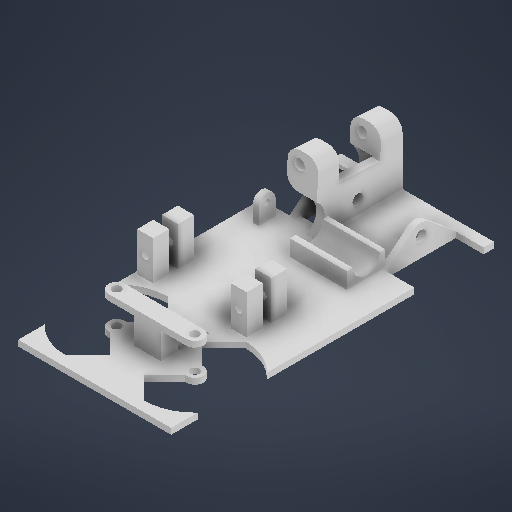
# Autodesk Inventor part: Рама
Saved by Autodesk Inventor 2026.2 (Build 302298000, 298)
## iProperties
Created: 2026-02-19
Part Number: Рама
Material: Типовые
Document SubType Name: Modeling
Designer: Leonid
Density: 1 g/cm^3
Appearance: По умолчанию
Author: Leonid
Autodesk Inventor part; units mm, degrees
ref_plane "XZ Plane" through (0, 0, 0) normal (0, 1, 0) x (-1, 0, 0)
ref_plane "XY Plane" through (0, 0, 0) normal (0, 0, 1) x (1, 0, 0)
sketch "Эскиз1" plane through (0, 0, 0) normal (0, 1, 0) x (-1, 0, 0)
  line L0 (-22.5, -47.5) -> (22.5, -47.5)
  line L1 (22.5, -47.5) -> (22.5, 14.5)
  line L2 (22.5, 47.5) -> (-22.5, 47.5)
  line L3 (-22.5, 47.5) -> (-22.5, 44.5)
  line L4 (-22.5, -47.5) -> (22.5, 47.5) construction
  line L5 (22.5, -47.5) -> (-22.5, 47.5) construction
  line L6 (22.5, 29.5) -> (-22.5, 29.5) construction
  line L7 (-22.5, 44.5) -> (-22.5, 14.5)
  line L8 (-22.5, 14.5) -> (-22.5, -47.5)
  line L9 (22.5, 14.5) -> (22.5, 44.5)
  line L10 (22.5, 44.5) -> (22.5, 47.5)
  circle A0 centre (11.5, 29.5) radius 1.325
  line L11 (22.5, 44.5) -> (5, 44.5)
  line L12 (-22.5, 44.5) -> (-5, 44.5)
  arc A1 (11.5, 27) -> (11.5, 32) centre (11.5, 29.5) ccw
  line L13 (11.5, 32) -> (5, 32)
  circle A2 centre (-11.5, 29.5) radius 1.325
  arc A3 (-11.5, 32) -> (-11.5, 27) centre (-11.5, 29.5) ccw
  line L14 (-11.5, 32) -> (-5, 32)
  line L15 (11.5, 27) -> (-11.5, 27)
  line L16 (22.5, 14.5) -> (-22.5, 14.5)
  line L17 (5, 32) -> (5, 44.5)
  line L18 (-5, 32) -> (-5, 44.5)
  line L19 (-11.5, 44.5) -> (-5, 38)
  line L20 (-11.5, 44.5) -> (-2.3076, 44.5) construction
  line L21 (11.5, 44.5) -> (5, 38)
  line L22 (11.5, 44.5) -> (20.6924, 44.5) construction
  line L23 (5, 38) -> (11, 32)
  line L24 (-5, 38) -> (-11, 32)
  arc A4 (-11.5, 44.5) -> (-22.5, 39.698) centre (-11.5, 29.5) ccw
  arc A5 (22.5, 39.698) -> (11.5, 44.5) centre (11.5, 29.5) ccw
  arc A6 (-22.5, 19.302) -> (-11.5, 14.5) centre (-11.5, 29.5) ccw
  arc A7 (11.5, 14.5) -> (22.5, 19.302) centre (11.5, 29.5) ccw
  line L25 (-11.5, 44.5) -> (-11.5, 14.5) construction
  line L26 (11.5, 44.5) -> (11.5, 14.5) construction
  line L27 (-11, 27) -> (-5, 21)
  line L28 (-11, 27) -> (-2.5147, 27) construction
  line L29 (-5, 21) -> (-11.5, 14.5)
  line L30 (11.5, 14.5) -> (5, 21)
  line L31 (11.5, 14.5) -> (20.6924, 14.5) construction
  line L32 (5, 21) -> (11, 27)
  line L33 (-5.8, 8.55) -> (-10.55, 8.55)
  line L34 (-10.55, 8.55) -> (-10.55, 13.3)
  line L35 (-10.55, 13.3) -> (-5.8, 13.3)
  line L36 (-5.8, 13.3) -> (-5.8, 8.55)
  line L37 (16.95, 8.55) -> (21.7, 8.55)
  line L38 (21.7, 8.55) -> (21.7, 13.3)
  line L39 (21.7, 13.3) -> (16.95, 13.3)
  line L40 (16.95, 13.3) -> (16.95, 8.55)
  line L41 (-5.8, 1.3) -> (-10.55, 1.3)
  line L42 (-10.55, 1.3) -> (-10.55, 6.05)
  line L43 (-10.55, 6.05) -> (-5.8, 6.05)
  line L44 (-5.8, 6.05) -> (-5.8, 1.3)
  line L45 (16.95, 1.3) -> (21.7, 1.3)
  line L46 (21.7, 1.3) -> (21.7, 6.05)
  line L47 (21.7, 6.05) -> (16.95, 6.05)
  line L48 (16.95, 6.05) -> (16.95, 1.3)
  line L49 (22.5, -44.5) -> (-22.5, -44.5)
  line L50 (-22.5, -24.104) -> (-14.25, -24.104)
  line L51 (-14.25, -24.104) -> (-14.25, -44.5)
  line L52 (22.5, -24.104) -> (14.25, -24.104)
  line L53 (14.25, -24.104) -> (14.25, -44.5)
  line L54 (7, -25.63) -> (12.5, -25.63)
  line L55 (12.5, -25.63) -> (12.5, -42.974)
  line L56 (12.5, -42.974) -> (7, -42.974)
  line L57 (7, -42.974) -> (7, -25.63)
  line L58 (-7.8, 13.3) -> (16.95, 13.3)
  line L59 (16.95, 13.3) -> (16.95, -11.2)
  line L60 (16.95, -11.2) -> (-7.8, -11.2)
  line L61 (-7.8, -11.2) -> (-7.8, 13.3)
  line L62 (-4, 27) -> (4, 27)
  line L63 (4, 27) -> (4, 32)
  line L64 (4, 32) -> (-4, 32)
  line L65 (-4, 32) -> (-4, 27)
  line L66 (-4, 27) -> (4, 32) construction
  line L67 (4, 27) -> (-4, 32) construction
  line L68 (12.5, -34.302) -> (14.25, -34.302) construction
  point P0 (0, 0)
  point P1 (13.75, 44.5)
  point P2 (-12.5, -44.5)
  point P3 (-7.8, 1.3)
  point P4 (16.95, 1.3)
  point P5 (-7.8, 8.55)
  point P6 (-7.8, 6.05)
  point P7 (0, 29.5)
  point P8 (-4, 27)
  point P9 (4, 27)
  dimension "d0" = 45
  dimension "d6" = 3
  dimension "d7" = 2.65
  dimension "d8" = 11
  dimension "d14" = 2.65
  dimension "d15" = 11
  dimension "d16" = 2.5
  dimension "d19" = 10
  dimension "d20" = 12.5
  dimension "d22" = 95
  dimension "d23" = 12.5
  dimension "d25" = 23
  dimension "d26" = 45
  dimension "d27" = 135
  dimension "d29" = 23
  dimension "d30" = 45
  dimension "d31" = 135
  dimension "d37" = 0.5
  dimension "d38" = 32.25
  dimension "d39" = 22.75
  dimension "d40" = 4.75
  dimension "d42" = 5.95
  dimension "d43" = 32.25
  dimension "d44" = 22.75
  dimension "d45" = 4.75
  dimension "d46" = 2.5
  dimension "d60" = 20.3961
  dimension "d61" = 3
  dimension "d62" = 20.396
  dimension "d63" = 8.25
  dimension "d70" = 5.55
  dimension "d72" = 5.5
  dimension "d73" = 17.344
  dimension "d101" = 24.5
  dimension "d102" = 2
  dimension "d120" = 8
  dimension "d123" = 1.75
  constraints: 138 end point, 31 point on line, 23 perpendicular, 22 parallel, 17 horizontal, 12 point on circle, 11 equal length, 10 midpoint, 8 centre point, 6 coincident, 6 collinear, 6 tangent, 1 vertical
  measures "d0" distance of L2.end L2.start
  measures "d6" distance of L9.end L2.start
  measures "d7" diameter of A0
  measures "d8" distance from line of A0.centre L9
  measures "d14" diameter of A2
  measures "d15" distance from line of L7 A2.centre
  measures "d16" radius of A3
  measures "d19" distance between parallel lines of L18 L17
  measures "d20" distance between parallel lines of L16 L15
  measures "d22" distance between parallel lines of L0 L2
  measures "d23" vertical distance of L3.end L14.start
  measures "d25" distance of A2.centre A0.centre
  measures "d26" angle of L19 L20
  measures "d27" angle of L21 L22
  measures "d29" distance of L19.start L21.start
  measures "d30" angle of L27 L28
  measures "d31" angle of L31 L30
  measures "d37" distance of L15.start L32.end
  measures "d38" distance between parallel lines of L34 L38
  measures "d39" distance between parallel lines of L36 L40
  measures "d40" distance between parallel lines of L35 L33
  measures "d42" distance from line of L25.end L33
  measures "d43" distance between parallel lines of L42 L46
  measures "d44" distance between parallel lines of L44 L48
  measures "d45" distance between parallel lines of L43 L41
  measures "d46" distance between parallel lines of L33 L43
  measures "d60" distance of A6.start A4.end
  measures "d61" distance between parallel lines of L0 L49
  measures "d62" distance of L49.end L50.start
  measures "d63" distance of L50.start L50.end
  measures "d70" distance between parallel lines of L1 L40
  measures "d72" distance between parallel lines of L57 L55
  measures "d73" distance between parallel lines of L56 L54
  measures "d101" distance between parallel lines of L58 L60
  measures "d102" distance between parallel lines of L44 L61
  measures "d120" distance between parallel lines of L63 L65
  measures "d123" distance of L68.start L68.end
extrude "Выдавливание1" add sketch "Эскиз1" along normal blind 1.75 contours L8 L49 L1 L0 | L8 L16 L1 L52 L53 L49 L51 L50 | L7 A6 L16 | L16 A7 L9 | L29 L27 L15 L32 L30 L16 | L7 L12 A4 | A5 L11 L9 | L3 L2 L10 L11 L17 L13 A1 L15 L63 L64 L65 A3 L14 L18 L12 | L12 L18 L19 | L21 L17 L11 | L18 L14 L24 | L65 L64 L63 L15 | L23 L13 L17 | L36 L58 L40 L59 L48 L60 L61 L41 L44 L43 L33 | L33 L61 L35 L36 | L33 L34 L35 L61 | L61 L41 L42 L43 | L43 L44 L41 L61 | L39 L38 L37 L40 | L47 L46 L45 L48
extrude "Выдавливание3" add sketch "Эскиз1" along normal blind 13.25 contours L33 L61 L35 L36 | L33 L34 L35 L61 | L61 L41 L42 L43 | L43 L44 L41 L61 | L39 L38 L37 L40 | L47 L46 L45 L48
sketch "Эскиз3" plane through (10.55, 1.75, 1.3) normal (0, 0, -1) x (-1, 0, 0)
  line L0 (-11.95, 0) -> (33.05, 0) projected
  line L1 (0, 0) -> (0, 11.5) projected
  point P0 (10.55, -1.75)
  point P1 (2.375, 5.95)
  point P2 (29.875, 5.95)
  dimension "d49" = 27.5
  dimension "d50" = 5.95
  dimension "d51" = 2.375
  dimension "d52" = 5.95
  measures "d49" distance of point (29.875, 5.95) point (2.375, 5.95)
  measures "d50" distance from line of L0 point (2.375, 5.95)
  measures "d51" distance from line of L1 point (2.375, 5.95)
  measures "d52" distance from line of L0 point (29.875, 5.95)
hole "Отверстие1" at (8.175, 7.7, 1.3) at (-19.325, 7.7, 1.3) direction (0, 0, 1) diameter 2.1 end through all
sketch "Эскиз4" plane through (14.25, 0, -24.104) normal (1, 0, 0) x (0, 0, -1)
  line L0 (0, 1.75) -> (20.396, 1.75) projected
  circle A0 centre (10.198, 5.6) radius 1.575
  line L1 (10.198, 5.6) -> (10.198, 1.75) construction
  arc A1 (12.4201, 8.3041) -> (7.9759, 8.3041) centre (10.198, 5.6) ccw
  line L2 (0, 1.75) -> (7.9759, 8.3041)
  line L3 (12.4201, 8.3041) -> (20.396, 1.75)
  point P0 (-24.104, 0)
  dimension "d64" = 3.15
  dimension "d65" = 3.85
  dimension "d66" = 3.5
  constraints: 6 end point, 2 centre point, 2 point on circle, 2 tangent, 1 coincident, 1 midpoint, 1 vertical
  measures "d64" diameter of A0
  measures "d65" distance of L1.start L1.end
  measures "d66" radius of A1
extrude "Выдавливание4" add sketch "Эскиз4" against normal blind 1.75
mirror "Зеркальное отражение1" about plane through (0, 0, 0) normal (1, 0, 0) of "Выдавливание4"
ref_plane "РабПлоскость2" through (-9.85, 0, 0) normal (1, 0, 0) x (0, 1, 0)
sketch "Эскиз5" plane through (-9.85, 0, 0) normal (1, 0, 0) x (0, 1, 0)
  circle A0 centre (5.6, -34.302) radius 1.575 projected
  line L0 (1.75, -42.974) -> (1.75, -25.63) projected
  arc A1 (1.75, -42.974) -> (1.75, -25.63) centre (5.6, -34.302) ccw
  line L1 (21.7915, -29.2645) -> (12.7877, -28.7233)
  line L2 (12.7877, -28.7233) -> (12.0676, -40.7016)
  line L3 (12.0676, -40.7016) -> (21.0714, -41.2429)
  line L4 (21.0714, -41.2429) -> (21.7915, -29.2645)
  line L5 (21.0714, -41.2429) -> (12.7877, -28.7233) construction
  line L6 (5.6, -34.302) -> (21.4314, -35.2537) construction
  line L7 (0, 19.302) -> (0, -24.104) projected
  line L8 (1.75, 30.825) -> (1.75, 28.175) projected
  line L9 (1.75, 30.825) -> (1.75, 28.175) projected
  line L10 (1.75, 13.3) -> (1.75, 8.55) projected
  line L11 (1.75, 8.55) -> (1.75, 13.3) projected
  line L12 (1.75, 8.55) -> (1.75, 13.3) projected
  line L13 (1.75, 13.3) -> (1.75, 8.55) projected
  line L14 (1.75, 1.3) -> (1.75, 6.05) projected
  line L15 (1.75, 6.05) -> (1.75, 1.3) projected
  line L16 (1.75, 1.3) -> (1.75, 6.05) projected
  line L17 (1.75, 6.05) -> (1.75, 1.3) projected
  line L18 (1.75, -44.5) -> (1.75, -42.974) projected
  line L19 (1.75, -24.104) -> (1.75, 19.302) projected
  line L20 (1.75, 19.302) -> (1.75, 14.5) projected
  line L21 (1.75, 14.5) -> (1.75, 21) projected
  line L22 (1.75, 21) -> (1.75, 27) projected
  line L23 (1.75, 27) -> (1.75, 32) projected
  line L24 (1.75, 32) -> (1.75, 38) projected
  line L25 (1.75, 38) -> (1.75, 44.5) projected
  line L26 (1.75, 44.5) -> (1.75, 39.698) projected
  line L27 (1.75, 39.698) -> (1.75, 47.5) projected
  line L28 (1.75, 47.5) -> (1.75, 39.698) projected
  line L29 (1.75, 39.698) -> (1.75, 44.5) projected
  line L30 (1.75, 44.5) -> (1.75, 38) projected
  line L31 (1.75, 38) -> (1.75, 32) projected
  line L32 (1.75, 32) -> (1.75, 27) projected
  line L33 (1.75, 27) -> (1.75, 21) projected
  line L34 (1.75, 21) -> (1.75, 14.5) projected
  line L35 (1.75, 14.5) -> (1.75, 19.302) projected
  line L36 (1.75, 19.302) -> (1.75, -24.104) projected
  line L37 (1.75, -42.974) -> (1.75, -25.63) projected
  line L38 (1.75, -44.5) -> (1.75, -47.5) projected
  line L39 (1.75, -47.5) -> (1.75, -44.5) projected
  line L40 (8.3041, -32.0799) -> (1.75, -24.104) projected
  arc A2 (8.3041, -36.5241) -> (8.3041, -32.0799) centre (5.6, -34.302) ccw projected
  line L41 (8.3041, -36.5241) -> (1.75, -44.5) projected
  line L42 (1.75, -25.63) -> (1.75, -24.104) projected
  line L43 (1.75, -24.104) -> (1.75, -44.5) projected
  circle A3 centre (6.5, -19.3308) radius 4.51
  line L44 (16.9295, -34.9831) -> (17.8295, -20.0119)
  line L45 (6.5, -19.3308) -> (17.8295, -20.0119)
  circle A4 centre (6.5, -19.3308) radius 4
  line L46 (8.5, -13.5708) -> (1.75, -13.5708)
  line L47 (1.75, -25.0908) -> (8.5, -25.0908)
  line L48 (8.5, -13.5708) -> (8.5, -25.0908)
  line L49 (6.5, -13.5708) -> (6.5, -25.0908)
  arc A5 (6.5, -21.8308) -> (6.5, -16.8308) centre (6.5, -19.3308) ccw
  line L50 (6.5, -16.8308) -> (1.75, -16.8308)
  line L51 (6.5, -21.8308) -> (1.75, -21.8308)
  circle A6 centre (6.5, -19.3308) radius 0.8
  line L52 (16.5605, -41.122) -> (20.0542, -41.332)
  line L53 (20.0542, -41.332) -> (19.8426, -44.8511)
  line L54 (19.8426, -44.8511) -> (16.349, -44.6411)
  line L55 (16.349, -44.6411) -> (16.5605, -41.122)
  line L56 (17.2986, -28.8442) -> (17.6705, -22.6571)
  line L57 (17.6705, -22.6571) -> (21.1642, -22.8672)
  line L58 (21.1642, -22.8672) -> (20.7923, -29.0542)
  line L59 (20.7923, -29.0542) -> (17.2986, -28.8442)
  line L60 (18.8708, -28.9387) -> (19.2427, -22.7516)
  line L61 (18.1327, -41.2165) -> (17.9211, -44.7356)
  line L62 (17.6705, -22.6571) -> (10.8765, -22.2487)
  line L63 (17.2986, -28.8442) -> (13.1812, -28.5966)
  line L64 (10.8765, -22.2487) -> (10.8765, -26.4163)
  line L65 (16.5605, -41.122) -> (12.4431, -40.8745)
  line L66 (1.75, -47.5) -> (19.6834, -47.5)
  line L67 (19.6834, -47.5) -> (19.8426, -44.8511)
  line L68 (17.9211, -44.7356) -> (17.7549, -47.5)
  arc A7 (1.75, -21.5903) -> (10.8765, -22.2487) centre (6.5, -19.3308) ccw
  line L69 (1.75, -24.104) -> (1.75, 19.302) projected
  line L70 (12.4431, -40.8745) -> (12.0586, -40.8514)
  line L71 (12.0586, -40.8514) -> (12.0676, -40.7016)
  line L72 (13.1812, -28.5966) -> (12.7967, -28.5735)
  line L73 (12.7967, -28.5735) -> (12.7877, -28.7233)
  point P0 (0, 0)
  point P1 (13.297, -28.7539)
  point P2 (14.6988, -31.6116)
  point P3 (12.577, -40.7323)
  point P4 (1.75, -25.63)
  point P5 (6.5, -14.8208)
  point P6 (1.75, -13.5708)
  point P7 (6.5, -24.8566)
  point P8 (6.5, -23.8408)
  point P9 (6.5, -15.3308)
  point P10 (6.5, -23.3308)
  point P11 (1.75, -16.8308)
  point P12 (1.75, -21.8308)
  point P13 (2.705, -43.3378)
  point P14 (1.8721, -21.8308)
  dimension "d38" = 32.25
  dimension "d78" = 11.35
  dimension "d80" = 9.02
  dimension "d124" = 12
  dimension "d125" = 9.02
  dimension "d126" = 4.75
  dimension "d127" = 1
  dimension "d129" = 11.35
  dimension "d130" = 8
  dimension "d131" = 1.25
  dimension "d132" = 2
  dimension "d137" = 2.5
  dimension "d142" = 1.6
  dimension "d143" = 0.15
  dimension "d144" = 0.15
  dimension "d145" = 2.65
  dimension "d146" = 3.5
  dimension "d148" = 1.575
  dimension "d151" = 0.75
  constraints: 70 end point, 16 point on line, 15 perpendicular, 10 collinear, 9 point on circle, 6 centre point, 5 coincident, 5 parallel, 3 midpoint, 2 horizontal, 2 vertical, 1 tangent, 2 other
  measures "d78" distance of A0.centre L44.start
  measures "d80" distance of L2.end L3.end
  measures "d124" distance between parallel lines of L3 L1
  measures "d125" diameter of A3
  measures "d126" distance from line of L45.start L19
  measures "d129" distance of L45.start L44.end
  measures "d130" diameter of A4
  measures "d131" distance edge to line of A3 L46
  measures "d132" distance between parallel lines of L49 L48
  measures "d137" radius of A5
  measures "d142" diameter of A6
  measures "d143" distance between parallel lines of L52 L3
  measures "d144" distance between parallel lines of L1 L59
  measures "d145" distance between parallel lines of L57 L45
  measures "d146" distance between parallel lines of L56 L58
  measures "d148" distance between parallel lines of L44 L60
  measures "d151" radial gap between concentric circles of A3 A7
extrude "Выдавливание12" add sketch "Эскиз1" along normal blind 9.45 contours L65 L64 L63 L15
ref_plane "РабПлоскость4" through (-22.5, 0, 17.8) normal (0, 0, 1) x (1, 0, 0)
sketch "Эскиз7" plane through (-22.5, 0, 17.8) normal (0, 0, 1) x (1, 0, 0)
  circle A0 centre (22.5, 8) radius 7.5
  line L0 (0, 1.75) -> (45, 1.75) projected
  line L1 (22.5, 1.75) -> (22.5, 8) construction
  point P0 (22.5, 0)
  point P1 (26.6458, 1.75)
  point P2 (18.3542, 1.75)
  dimension "d110" = 15
  dimension "d111" = 6.25
  constraints: 2 end point, 1 centre point, 1 midpoint, 1 vertical
  measures "d110" diameter of A0
  measures "d111" distance of L1.start L1.end
extrude "Выдавливание15" cut sketch "Эскиз7" along normal blind 8.75 contours L0 A0 picked at (21.6394, 1.4861)
sketch "Эскиз8" plane through (0, 9.45, 0) normal (0, 1, 0) x (1, 0, 0)
  arc A0 (11.5, -32) -> (11.5, -27) centre (11.5, -29.5) ccw projected
  line L0 (-11.5, -27) -> (11.5, -27) projected
  arc A1 (-11.5, -27) -> (-11.5, -32) centre (-11.5, -29.5) ccw projected
  line L1 (-11.5, -32) -> (-11, -32) construction
  line L2 (-11.5, -32) -> (11.5, -32)
  circle A2 centre (-11.5, -29.5) radius 1.325 projected
  circle A3 centre (11.5, -29.5) radius 1.325 projected
  point P0 (0, 0)
  constraints: 2 end point, 1 horizontal, 1 tangent
extrude "Выдавливание16" add sketch "Эскиз8" along normal blind 1.75
extrude "Выдавливание17" add sketch "Эскиз5" along normal blind 23 contours L42 L47 L40 A1 | L40 L47 A1 | L42 L40 L47 | L47 L40 L19 L51 A7 L49 A1 | L19 A7 L51 | A7 L51 A3 L49 | L19 L50 A3 L51 A7 | A3 L51 A4 L49 | L19 L46 L49 A3 L50 | A3 L50 A4 L51 | A3 L49 A4 L50
extrude "Выдавливание18" cut sketch "Эскиз5" along normal blind 6.2 contours L42 L47 L40 A1 | L40 L47 A1 | L42 L40 L47 | L47 L40 L19 L51 A7 L49 A1 | L19 A7 L51 | A7 L51 A3 L49 | L19 L50 A3 L51 A7 | A3 L51 A4 L49 | L19 L46 L49 A3 L50 | A3 L50 A4 L51 | A3 L49 A4 L50
extrude "Выдавливание19" add sketch "Эскиз5" against normal blind 7.95 contours L19 A7 L51 | L19 L50 A3 L51 A7 | A3 L50 A4 L51 | A4 L50 L49 A6 L51 | L49 A6 L45 L48 A5 | L48 L45 A5 | A5 L48 L45 A6 L49 | L45 L48 A5
extrude "Выдавливание20" cut sketch "Эскиз5" against normal blind 6.2 contours L19 A7 L51 | L19 L50 A3 L51 A7 | A3 L50 A4 L51 | A4 L50 L49 A6 L51 | L49 A6 L45 L48 A5 | L48 L45 A5 | A6 L49 | L49 L45 A6 | A5 L48 L45 A6 L49 | L45 L48 A5 | L49 A6 L45
extrude "Выдавливание21" add sketch "Эскиз5" along normal mid plane 7 contours A1 L65 L55 L54 L68 L66 L38 L41 | L52 L61 L54 L55 | L68 L54 L67 L66 | L52 L53 L54 L61 | A1 L64 L62 L44 L63 | L44 L57 L60 L59 | L60 L57 L58 L59
extrude "Выдавливание22" add sketch "Эскиз5" along normal blind 5.5 contours L0 A1 L40 A2 L41 | A1 L41 L18 | L42 L47 L40 A1 | L41 A2 L40 A1 L47 L72 L73 L2 L71 L70 | A1 L65 L55 L54 L68 L66 L38 L41 | L40 L47 A1 | L42 L40 L47 | L47 L40 L19 L51 A7 L49 A1 | A1 L49 L47 | L52 L61 L54 L55 | L68 L54 L67 L66 | L49 A7 L48 L47 A1 | A1 L47 L49 | L52 L53 L54 L61 | L47 L48 A7 L64 A1 | A1 L64 L62 L44 L63 | L44 L57 L60 L59 | L60 L57 L58 L59
extrude "Выдавливание23" cut sketch "Эскиз5" along normal blind 3 contours L0 A1 L40 A2 L41 | L42 L47 L40 A1 | L41 A2 L40 A1 L47 L72 L73 L2 L71 L70 | L40 L47 A1 | L42 L40 L47 | L47 L40 L19 L51 A7 L49 A1 | A1 L49 L47 | L49 A7 L48 L47 A1 | A1 L47 L49 | L47 L48 A7 L64 A1
sketch "Эскиз9" plane through (-13.35, 21.1642, -22.8672) normal (0, 0.0600072, 0.9981979) x (1, 0, 0)
  point P0 (13.35, -22.4983)
  point P1 (3.5, -3.5)
  point P2 (3.5, -3.5)
  point P3 (3.5, -3.5)
  point P4 (3.5, -3.5)
hole "Отверстие3" at (-9.85, 17.6705, -22.6571) direction (0, -0.0600072, -0.9981979) diameter 3.15 end through all
fillet "Сопряжение2" radius 3.5 5 edges at (-13.35, 19.8688, -44.416) (-13.35, 20.9783, -25.9607) (-13.35, 10.8765, -24.3325) (-4.35, 20.9783, -25.9607) (-4.35, 19.8688, -44.416)
